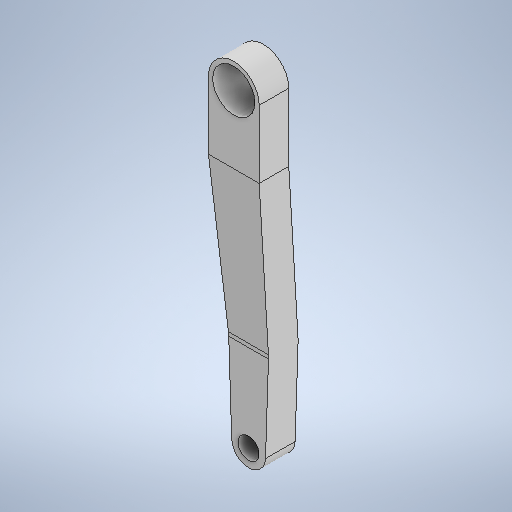
# Autodesk Inventor part: 47
Saved by Autodesk Inventor 2025.1 (Build 291241000, 241)
## iProperties
Created: 2024-09-17
Part Number: 47
Material: Generisch
Document SubType Name: Modeling
Designer: ffogue
Density: 1 g/cm^3
Appearance: Vorgabe
Author: ffogue
Autodesk Inventor part; units mm, degrees
ref_plane "YZ Plane" through (0, 0, 0) normal (1, 0, 0) x (0, 1, 0)
ref_plane "XZ Plane" through (0, 0, 0) normal (0, 1, 0) x (-1, 0, 0)
ref_plane "XY Plane" through (0, 0, 0) normal (0, 0, 1) x (1, 0, 0)
sketch "Sketch19" plane through (0, 0, 0) normal (1, 0, 0) x (0, 1, 0)
  line L0 (0, 0) -> (0, -22)
  line L1 (0, -22) -> (3.4577, -59.4814)
  line L2 (3.5, -60.4) -> (3.5, -85)
  line L3 (3.5, -85) -> (10.5, -85)
  line L4 (10.5, -85) -> (10.5, -60.4)
  line L5 (10.4577, -59.4814) -> (7, -22)
  line L6 (7, -22) -> (7, 0)
  line L7 (7, 0) -> (0, 0)
  arc A0 (3.5, -60.4) -> (3.4577, -59.4814) centre (-6.5, -60.4) ccw
  arc A1 (10.5, -60.4) -> (10.4577, -59.4814) centre (0.5, -60.4) ccw
  point P0 (10.4894, -59.9402)
  dimension "d79" = 10
  dimension "d80" = 10
  dimension "d82" = 7
  dimension "d83" = 3.5
  dimension "d84" = 24.6
  dimension "d85" = 22
  dimension "d86" = 37.9402
  constraints: 16 end point, 5 point on circle, 4 tangent, 3 parallel, 3 perpendicular, 2 centre point, 2 horizontal alignment, 1 vertical
  measures "d79" radius of A0
  measures "d80" radius of A1
  measures "d82" distance of L6.end L0.start
  measures "d83" distance between parallel lines of L0 L2
  measures "d84" distance of L3.end L4.end
  measures "d85" distance of L5.end L6.end
  measures "d86" vertical distance of point (10.489, -59.94) L5.end
extrude "Extrusion7" add sketch "Sketch19" along normal blind 12
sketch "Sketch20" plane through (0, 7, 0) normal (0, 1, 0) x (1, 0, 0)
  circle A0 centre (6, 6) radius 6
  line L0 (0, 0) -> (12, 0) projected
  line L1 (0, 0) -> (12, 0) projected
  line L2 (0, 0) -> (0, 6)
  line L3 (0, 0) -> (0, 22) projected
  line L4 (12, 0) -> (12, 6)
  point P0 (6, 0)
  point P1 (6, 0)
  dimension "d89" = 12
  constraints: 4 end point, 3 point on circle, 2 midpoint, 1 centre point, 1 point on line, 1 tangent, 1 vertical alignment
  measures "d89" diameter of A0
extrude "Extrusion8" cut sketch "Sketch20" against normal blind 12 contours L4 L0 A0 | A0 L0 L2
sketch "Sketch21" plane through (0, 10.5, -60.4) normal (0, 1, 0) x (1, 0, 0)
  circle A0 centre (6, 20.6) radius 4
  line L0 (0, 24.6) -> (12, 24.6) projected
  arc A1 (0, -54.4) -> (12, -54.4) centre (6, -54.4) ccw projected
  line L1 (12, -38.4) -> (12, -54.4) projected
  line L2 (0, -38.4) -> (12, -38.4) projected
  line L3 (0, -38.4) -> (0, -54.4) projected
  line L4 (0, -38.4) -> (2.0023, 20.7354)
  line L5 (12, -38.4) -> (12, -0.9186) projected
  line L6 (12, -38.4) -> (9.9977, 20.7354)
  line L7 (0, 24.6) -> (0, 0) projected
  line L8 (0, -38.4) -> (0, 24.6)
  line L9 (0, 24.6) -> (6, 24.6)
  line L10 (6, 24.6) -> (12, 24.6)
  line L11 (12, 0) -> (12, 24.6) projected
  line L12 (12, 24.6) -> (12, -38.4)
  point P0 (0, -60.4)
  point P1 (12, 0)
  dimension "d93" = 8
  constraints: 12 end point, 4 tangent, 3 collinear, 3 point on circle, 2 midpoint, 1 centre point, 1 perpendicular, 1 vertical alignment
  measures "d93" diameter of A0
extrude "Extrusion9" cut sketch "Sketch21" against normal up to surface (10.5 mm away) contours A0 L0 L11 L12 L5 L6 | L4 L8 L7 L0 A0
sketch "Sketch22" plane through (6, 7, -6) normal (0, 1, 0) x (1, 0, 0)
  arc A0 (-6, 0) -> (6, 0) centre (0, 0) ccw projected
  point P0 (-6, -6)
  constraints: 1 coincident
hole "Hole1" at (6, 7, -6) direction (0, -1, 0) diameter 10 end through all
sketch "Sketch23" plane through (6, 10.5, -81) normal (0, 1, 0) x (1, 0, 0)
  arc A0 (3.9977, 0.1354) -> (-3.9977, 0.1354) centre (0, 0) ccw projected
  point P0 (-6, -81)
  constraints: 1 coincident
hole "Hole2" at (6, 10.5, -81) direction (0, -1, 0) diameter 5 end through all
fillet "Fillet1" radius 10 1 edges at (6, 7, -22)
body "Solid2"
